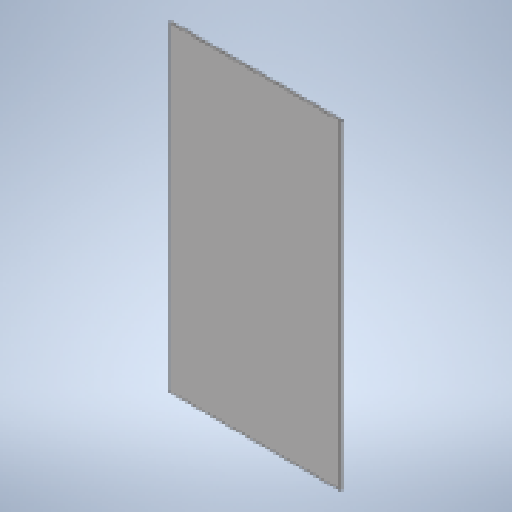
# Autodesk Inventor part: DF1.04 Wall face v2.0
Saved by Autodesk Inventor 2026.3 (Build 303398000, 398)
## iProperties
Created: 2023-08-31
Part Number: DF1.04 Wall face v2.0
Material: Generic
Document SubType Name: Sheet Metal
Designer: admin
Density: 1 g/cm^3
Sheet Metal Rule: Default_mm
Appearance: Default
Flat Pattern Width: 115 cm
Flat Pattern Length: 214 cm
Flat Pattern Area: 24610 cm^2
Sheet Metal Width: 1150,000 mm
Sheet Metal Length: 2140,000 mm
Sheet Metal Area: 2461000,000 mm^2
Author: admin
Autodesk Inventor part; units mm, degrees
ref_plane "YZ Plane" through (0, 0, 0) normal (1, 0, 0) x (0, 1, 0)
ref_plane "XZ Plane" through (0, 0, 0) normal (0, 1, 0) x (-1, 0, 0)
ref_plane "XY Plane" through (0, 0, 0) normal (0, 0, 1) x (1, 0, 0)
sketch "Sketch1" plane through (0, 0, 0) normal (0, 0, 1) x (1, 0, 0)
  line L0 (-575, -1070) -> (575, -1070)
  line L1 (575, -1070) -> (575, 1070)
  line L2 (575, 1070) -> (-575, 1070)
  line L3 (-575, 1070) -> (-575, -1070)
  line L4 (-575, -1070) -> (575, 1070) construction
  line L5 (575, -1070) -> (-575, 1070) construction
  point P0 (0, 0)
  dimension "d1" = 1150
  dimension "d2" = 2140
  constraints: 12 end point, 2 midpoint, 2 parallel, 1 horizontal, 1 perpendicular
  measures "d1" distance of L0.start L0.end
  measures "d2" distance of L2.end L0.start
extrude "Plate1" add sketch "Sketch1" along normal blind 10
equation "\"d0\" = Thickness"
equation "\"BendReliefDepth\" = 0.5 * Thickness"
equation "\"Thickness\" = 10"
body "Solid1"
